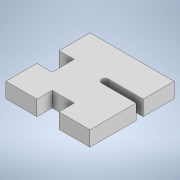
# Autodesk Inventor part: SupportV2
Saved by Autodesk Inventor 2020 (Build 240168000, 168)
## iProperties
Created: 2019-11-07
Part Number: SupportV2
Material: Générique
Document SubType Name: Modeling
Designer: erwan
Density: 1 g/cm^3
Appearance: Par défaut
Author: erwan
Autodesk Inventor part; units mm, degrees
ref_plane "YZ Plane" through (0, 0, 0) normal (1, 0, 0) x (0, 1, 0)
ref_plane "XZ Plane" through (0, 0, 0) normal (0, 1, 0) x (-1, 0, 0)
ref_plane "XY Plane" through (0, 0, 0) normal (0, 0, 1) x (1, 0, 0)
sketch "Esquisse1" plane through (0, 0, 0) normal (0, 1, 0) x (-1, 0, 0)
  line L0 (0, -122) -> (0, -77)
  line L1 (0, -77) -> (50, -77)
  arc A0 (50, -77) -> (50, -67) centre (50, -72) ccw
  line L2 (50, -67) -> (0, -67)
  line L3 (0, 0) -> (0, -67)
  line L4 (122, -122) -> (122, -77)
  line L5 (122, -77) -> (100, -77)
  line L6 (100, -77) -> (100, -45)
  line L7 (100, -45) -> (122, -45)
  line L8 (122, -45) -> (122, 0)
  line L9 (122, 0) -> (77, 0)
  line L10 (77, 0) -> (77, -22)
  line L11 (77, -22) -> (45, -22)
  line L12 (45, -22) -> (45, 0)
  line L13 (45, 0) -> (0, 0)
  line L14 (122, -122) -> (0, -122)
  dimension "d0" = 122
  dimension "d1" = 122
  dimension "d2" = 45
  dimension "d3" = 50
  dimension "d10" = 45
  dimension "d11" = 22
  dimension "d12" = 32
  dimension "d13" = 45
  dimension "d14" = 22
  dimension "d15" = 32
  constraints: 30 end point, 10 perpendicular, 2 point on circle, 2 point on line, 2 vertical, 1 centre point, 1 horizontal
  measures "d0" distance of L4.start L0.start
  measures "d1" distance of L8.end L4.start
  measures "d2" distance of L0.start L0.end
  measures "d3" distance of L0.end L1.end
  measures "d10" distance of L4.start L4.end
  measures "d11" distance of L4.end L5.end
  measures "d12" distance of L5.end L6.end
  measures "d13" distance of L8.end L9.end
  measures "d14" distance of L9.end L10.end
  measures "d15" distance of L10.end L11.end
extrude "Extrusion1" add sketch "Esquisse1" along normal blind 22
